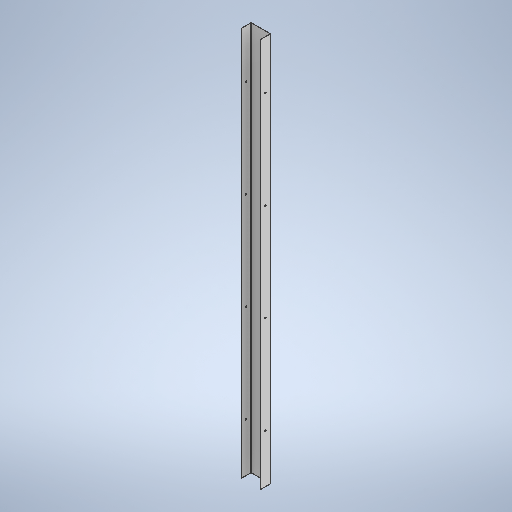
# Autodesk Inventor part: Beam_A1
Saved by Autodesk Inventor 2025.2 (Build 292293000, 293)
## iProperties
Created: 2025-03-13
Part Number: Beam_A1
Material: Generic
Document SubType Name: Sheet Metal
Designer: Andreas' PC
Density: 1 g/cm^3
Sheet Metal Rule: Default_mm
Appearance: Default
Author: Andreas' PC
Autodesk Inventor part; units mm, degrees
ref_plane "YZ Plane" through (0, 0, 0) normal (1, 0, 0) x (0, 1, 0)
ref_plane "XZ Plane" through (0, 0, 0) normal (0, 1, 0) x (-1, 0, 0)
ref_plane "XY Plane" through (0, 0, 0) normal (0, 0, 1) x (1, 0, 0)
sketch "Sketch1" plane through (0, 0, 0) normal (0, 0, 1) x (1, 0, 0)
  line L0 (0, 0) -> (50, 0)
  line L1 (50, 0) -> (50, 1000)
  line L2 (50, 1000) -> (0, 1000)
  line L3 (0, 1000) -> (0, 0)
  dimension "d0" = 50
  dimension "d1" = 1000
  measures "d0" distance of L2.end L1.end
  measures "d1" distance of L1.end L0.end
extrude "Plate1" add sketch "Sketch1" along normal blind 0.5
sketch "Sketch2" plane through (49.5, 1000, 0) normal (1, 0, 0) x (0, 1, 0)
  line L0 (-1000, 0) -> (0, 0)
  line L1 (0, 0) -> (0, 25)
  line L2 (0, 25) -> (-1000, 25)
  line L3 (-1000, 25) -> (-1000, 0)
  constraints: 6 end point, 1 horizontal, 1 perpendicular, 1 vertical
edge flange "Flange1" height 25 angle 90 thickness 0.5 bend radius 0.5 thickness toward (1, 0, 0) relief straight relief width 0.5 relief depth 0.25 edges at (50, 500, 0.5) wall of the first edge with corners at (49.5, 0, 0) (49.5, 1000, 0) (49.5, 1000, 25) (49.5, 0, 25)
bend "Bend1"
corner "Corner1"
sketch "Sketch3" plane through (0.5, 0, 0) normal (-1, 0, 0) x (0, -1, 0)
  line L0 (-1000, 0) -> (0, 0)
  line L1 (0, 0) -> (0, 25)
  line L2 (0, 25) -> (-1000, 25)
  line L3 (-1000, 25) -> (-1000, 0)
  constraints: 6 end point, 1 horizontal, 1 perpendicular, 1 vertical
edge flange "Flange2" height 25 angle 90 thickness 0.5 bend radius 0.5 thickness toward (-1, 0, 0) relief straight relief width 0.5 relief depth 0.25 edges at (0, 500, 0.5) wall of the first edge with corners at (0.5, 1000, 0) (0.5, 0, 0) (0.5, 0, 25) (0.5, 1000, 25)
bend "Bend2"
corner "Corner2"
sketch "Sketch4" plane through (0, 0, 25) normal (-1, 0, 0) x (0, 0, 1)
  circle A0 centre (-11.5, 125) radius 2
  line L0 (0, 0) -> (-24, 0) projected
  circle A1 centre (-11.5, 375) radius 2
  line L1 (-24, 1000) -> (-24, 0) projected
  circle A2 centre (-11.5, 625) radius 2
  circle A3 centre (-11.5, 875) radius 2
  line L2 (-24, 1000) -> (0, 1000) projected
  point P0 (-25, 0)
  dimension "d23" = 4
  dimension "d24" = 125
  dimension "d25" = 4
  dimension "d26" = 250
  dimension "d27" = 12.5
  dimension "d28" = 12.5
  dimension "d29" = 4
  dimension "d30" = 250
  dimension "d31" = 12.5
  dimension "d32" = 4
  dimension "d33" = 250
  dimension "d34" = 12.5
  dimension "d35" = 125
  constraints: 4 centre point
  measures "d23" diameter of A0
  measures "d24" distance from line of L0 A0.centre
  measures "d25" diameter of A1
  measures "d26" distance of A0.centre A1.centre
  measures "d27" distance from line of L1 A0.centre
  measures "d28" distance from line of L1 A1.centre
  measures "d29" diameter of A2
  measures "d30" distance of A1.centre A2.centre
  measures "d31" distance from line of L1 A2.centre
  measures "d32" diameter of A3
  measures "d33" distance of A3.centre A2.centre
  measures "d34" distance from line of L1 A3.centre
  measures "d35" distance from line of L2 A3.centre
hole "Hole1" at (0, 375, 13.5) at (0, 625, 13.5) at (0, 125, 13.5) at (0, 875, 13.5) direction (1, 0, 0) diameter 4 end through all
equation "\"d0\" = A_width"
equation "\"d1\" = A_length"
equation "\"d23\" = rivet_diameter"
equation "\"d24\" = 0.5 * rivet_displacement"
equation "\"d25\" = rivet_diameter"
equation "\"d26\" = rivet_displacement"
equation "\"d27\" = 0.25 * A_width"
equation "\"d28\" = 0.25 * A_width"
equation "\"d29\" = rivet_diameter"
equation "\"d30\" = rivet_displacement"
equation "\"d31\" = 0.25 * A_width"
equation "\"d32\" = rivet_diameter"
equation "\"d33\" = rivet_displacement"
equation "\"d34\" = 0.25 * A_width"
equation "\"d36\" = rivet_diameter"
equation "\"d41\" = Thickness"
equation "\"d2\" = Thickness"
equation "\"d3\" = BendReliefWidth"
equation "\"d4\" = BendReliefDepth"
equation "\"d5\" = MinimumRemnant"
equation "\"d6\" = TransitionRadius"
equation "\"d7\" = 0.5 * A_width"
equation "\"d9\" = BendRadius"
equation "\"d10\" = CornerReliefSize"
equation "\"d11\" = GapSize"
equation "\"d12\" = JacobiRadiusSize"
equation "\"d13\" = BendReliefWidth"
equation "\"d14\" = BendReliefDepth"
equation "\"d15\" = MinimumRemnant"
equation "\"d16\" = TransitionRadius"
equation "\"d17\" = 0.5 * A_width"
equation "\"d19\" = BendRadius"
equation "\"d20\" = CornerReliefSize"
equation "\"d21\" = GapSize"
equation "\"d22\" = JacobiRadiusSize"
equation "\"BendRadius\" = Thickness"
equation "\"BendReliefWidth\" = Thickness"
equation "\"BendReliefDepth\" = 0.5 * Thickness"
equation "\"CornerReliefSize\" = 4 * Thickness"
equation "\"MinimumRemnant\" = 2 * Thickness"
equation "\"TransitionRadius\" = BendRadius"
equation "\"JacobiRadiusSize\" = BendRadius"
equation "\"GapSize\" = Thickness"
equation "\"A_length\" = 1000"
equation "\"A_width\" = 50"
equation "\"l___________\" = 0"
equation "\"l__________\" = 0"
equation "\"l_________\" = 0"
equation "\"rivet_diameter\" = 4"
equation "\"rivet_displacement\" = 250"
equation "\"l________\" = 0"
equation "\"Thickness\" = 0.5"
body "Solid1"
